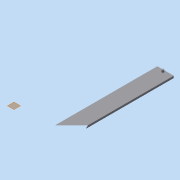
# Autodesk Inventor part: sideframe
Saved by Autodesk Inventor 2016 (Build 200138000, 138)
## iProperties
Created: 2017-03-05
Part Number: sideframe
Material: Generic
Document SubType Name: Modeling
Designer: Errrm
Density: 1 g/cm^3
Appearance: Default
Author: Errrm
Autodesk Inventor part; units mm, degrees
ref_plane "YZ Plane" through (0, 0, 0) normal (1, 0, 0) x (0, 1, 0)
ref_plane "XZ Plane" through (0, 0, 0) normal (0, 1, 0) x (-1, 0, 0)
ref_plane "Work Plane1" through (0, 0, 18.5) normal (0, 0, 1) x (1, 0, 0)
sketch "Sketch1" plane through (0, 0, 18.5) normal (0, 0, 1) x (1, 0, 0)
  line L0 (119.7216, 316.2246) -> (169.7216, 316.2246)
  line L1 (169.7216, 316.2246) -> (169.7216, -13.7754)
  line L2 (169.7216, -13.7754) -> (119.7216, -13.7754)
  line L3 (119.7216, -13.7754) -> (119.7216, 316.2246)
  point P0 (0, 0)
  dimension "d1" = 330
  dimension "d4" = 50
  constraints: 8 end point, 2 parallel, 1 horizontal, 1 perpendicular
  measures "d1" distance of L0.end L1.end
  measures "d4" distance of L0.start L0.end
extrude "Extrusion1" add sketch "Sketch1" along normal blind 6
sketch "Sketch2" plane through (0, 0, 24.5) normal (0, 0, 1) x (1, 0, 0)
  circle A0 centre (142.8603, 309.8004) radius 3.2743
  point P0 (0, 0)
  constraints: 1 centre point
extrude "Extrusion2" add sketch "Sketch2" along normal blind 6
body "Solid1"
